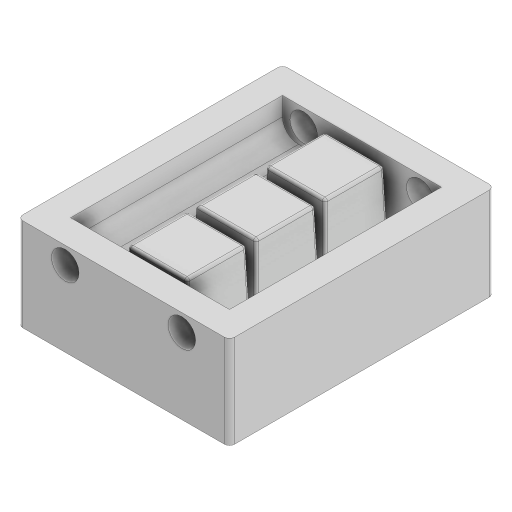
# Autodesk Inventor part: Mould_3 wells
Saved by Autodesk Inventor 2023 (Build 270158000, 158)
## iProperties
Created: 2026-05-27
Part Number: Mould_3 wells
Material: Generic
Document SubType Name: Modeling
Designer: ferrerx
Density: 1 g/cm^3
Appearance: Default
Author: ferrerx
Autodesk Inventor part; units mm, degrees
ref_plane "YZ Plane" through (0, 0, 0) normal (1, 0, 0) x (0, 1, 0)
ref_plane "XZ Plane" through (0, 0, 0) normal (0, 1, 0) x (-1, 0, 0)
ref_plane "XY Plane" through (0, 0, 0) normal (0, 0, 1) x (1, 0, 0)
sketch "Sketch1" plane through (0, 0, 0) normal (0, 1, 0) x (-1, 0, 0)
  line L0 (-20, 25) -> (20, 25)
  line L1 (20, 25) -> (20, -25)
  line L2 (20, -25) -> (-20, -25)
  line L3 (-20, -25) -> (-20, 25)
  line L4 (-20, 25) -> (20, -25) construction
  line L5 (20, 25) -> (-20, -25) construction
  point P0 (0, 0)
  dimension "d0" = 50
  dimension "d1" = 40
  constraints: 12 end point, 2 midpoint, 2 parallel, 1 horizontal, 1 perpendicular
  measures "d0" distance of L0.end L1.end
  measures "d1" distance of L0.start L0.end
extrude "Extrusion1" add sketch "Sketch1" along normal blind 5
sketch "Sketch3" plane through (0, 5, 0) normal (0, 1, 0) x (1, 0, 0)
  line L0 (6, -6) -> (-6, -6)
  line L1 (-6, -6) -> (-6, 6)
  line L2 (-6, 6) -> (6, 6)
  line L3 (6, 6) -> (6, -6)
  line L4 (6, -6) -> (-6, 6) construction
  line L5 (-6, -6) -> (6, 6) construction
  point P0 (0, 0)
  dimension "d4" = 12
  dimension "d5" = 12
  constraints: 12 end point, 2 midpoint, 2 parallel, 1 horizontal, 1 perpendicular
  measures "d4" distance of L1.end L2.end
  measures "d5" distance of L0.end L1.end
extrude "Extrusion2" add sketch "Sketch3" along normal blind 12 draft -2
pattern_linear "Rectangular Pattern1" count 3 spacing 13 along (0, 0, -1) of "Extrusion2" first direction both ways yes
sketch "Sketch4" plane through (0, 5, 0) normal (0, 1, 0) x (1, 0, 0)
  line L0 (20, 25) -> (-20, 25) projected
  line L1 (20, -25) -> (-20, -25)
  line L2 (-20, -25) -> (-20, 25)
  line L3 (-20, 25) -> (20, 25)
  line L4 (20, 25) -> (20, -25)
  line L5 (20, -25) -> (-20, 25) construction
  line L6 (-20, -25) -> (20, 25) construction
  line L7 (15, -20) -> (-15, -20)
  line L8 (-15, -20) -> (-15, 20)
  line L9 (-15, 20) -> (15, 20)
  line L10 (15, 20) -> (15, -20)
  line L11 (15, -20) -> (-15, 20) construction
  line L12 (-15, -20) -> (15, 20) construction
  point P0 (0, 0)
  dimension "d11" = 5
  dimension "d12" = 5
  constraints: 24 end point, 4 midpoint, 4 parallel, 2 horizontal, 2 perpendicular
  measures "d11" distance between parallel lines of L2 L8
  measures "d12" distance between parallel lines of L1 L7
extrude "Extrusion3" add sketch "Sketch4" along normal blind 12.5
sketch "Sketch5" plane through (0, 5, 0) normal (0, 1, 0) x (1, 0, 0)
  line L0 (-15, 20) -> (-15, -20) projected
  line L1 (15, 20) -> (-15, 20) projected
  line L2 (-15, -20) -> (-7, -20)
  line L3 (-7, -20) -> (-7, 20)
  line L4 (-7, 20) -> (-15, 20)
  line L5 (-15, 20) -> (-15, -20)
  line L6 (15, 20) -> (15, -20) projected
  line L7 (15, -20) -> (7, -20)
  line L8 (7, -20) -> (7, 20)
  line L9 (7, 20) -> (15, 20)
  line L10 (15, 20) -> (15, -20)
  point P0 (0, 0)
  point P1 (7, 20)
  dimension "d15" = 8
  dimension "d16" = 8
  constraints: 16 end point, 4 parallel, 2 horizontal, 2 perpendicular, 2 point on line
  measures "d15" distance between parallel lines of L6 L8
  measures "d16" distance between parallel lines of L0 L3
extrude "Extrusion4" add sketch "Sketch5" along normal blind 6
sketch "Sketch6" plane through (20, 0, -25) normal (0, 0, -1) x (-1, 0, 0)
  line L0 (5, 11) -> (13, 11) projected
  line L1 (9, 11) -> (9, 14.25) construction
  circle A0 centre (9, 14.25) radius 2.6
  line L2 (40, 17.5) -> (0, 17.5) projected
  line L3 (20, 17.5) -> (20, 0) construction
  circle A1 centre (31, 14.25) radius 2.6
  dimension "d19" = 5.2
  dimension "d20" = 3.25
  constraints: 4 end point, 2 centre point, 2 midpoint, 2 vertical, 1 coincident, 1 symmetric about line, 1 other
  measures "d19" diameter of A0
  measures "d20" distance of L1.start L1.end
extrude "Extrusion5" cut sketch "Sketch6" against normal blind 57.25
fillet "Fillet1" radius 3 4 edges at (7, 11, 0) (15, 11, 0) (-7, 11, 0) (-15, 11, 0)
fillet "Fillet2" radius 0.5 23 edges at (-5.7905, 11, -18.7905) (-5.7905, 11, -5.7905) (-5.7905, 11, 7.2095) (-5.7905, 11, 18.7905) (5.7905, 11, -18.7905) (5.7905, 11, -7.2095) (5.7905, 11, -5.7905) (5.7905, 11, 5.7905) (5.7905, 11, 7.2095) (5.7905, 11, 18.7905) (5.581, 17, 13) (0, 17, 7.419) (-5.581, 17, 13) (0, 17, 18.581) (0, 17, -5.581) (-5.581, 17, 0) (0, 17, 5.581) (5.581, 17, 0) (0, 17, -7.419) (-5.581, 17, -13) (0, 17, -18.581) (5.581, 17, -13) (-5.7905, 11, -7.2095)
fillet "Fillet3" radius 1 4 edges at (-20, 8.75, -25) (20, 8.75, -25) (-20, 8.75, 25) (20, 8.75, 25)
fillet "Fillet4" [suppressed]
body "Solid1"
